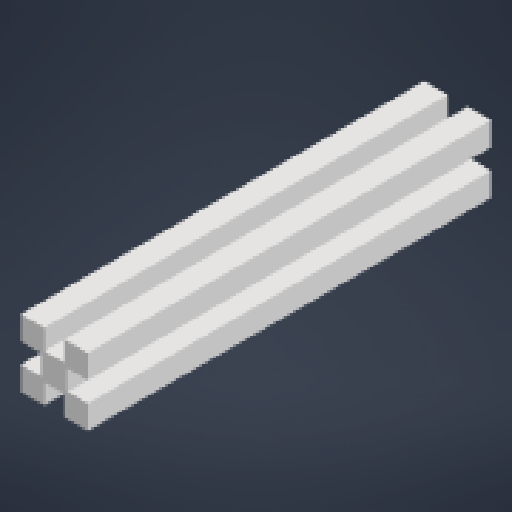
# Autodesk Inventor part: zbar
Saved by Autodesk Inventor 2025.1 (Build 291241020, 241B)
## iProperties
Created: 2024-09-23
Part Number: zbar
Material: Generic
Document SubType Name: Modeling
Designer: techn
Density: 1 g/cm^3
Appearance: Default
Author: techn
Autodesk Inventor part; units mm, degrees
ref_plane "YZ Plane" through (0, 0, 0) normal (1, 0, 0) x (0, 1, 0)
ref_plane "XZ Plane" through (0, 0, 0) normal (0, 1, 0) x (-1, 0, 0)
ref_plane "XY Plane" through (0, 0, 0) normal (0, 0, 1) x (1, 0, 0)
sketch "Sketch1" plane through (0, 0, 0) normal (0, 0, 1) x (1, 0, 0)
  line L0 (18, 7) -> (-162, 7) projected
  line L1 (-162, 0) -> (-162, 7) projected
  line L2 (18, 0) -> (-162, 0) projected
  line L3 (18, 7) -> (18, 0) projected
  line L4 (18, -6) -> (-162, -6) projected
  line L5 (-162, -13) -> (-162, -6) projected
  line L6 (-162, -13) -> (18, -13) projected
  line L7 (18, -6) -> (18, -13) projected
  line L8 (18, 0) -> (18, -6) projected
  line L9 (18, 7) -> (11, 7)
  line L10 (11, 7) -> (11, 0)
  line L11 (11, 0) -> (18, 0)
  line L12 (18, 0) -> (18, 7)
  line L13 (18, -6) -> (11, -6)
  line L14 (11, -6) -> (11, -13)
  line L15 (11, -13) -> (18, -13)
  line L16 (18, -13) -> (18, -6)
  line L17 (5, -13) -> (-2, -13)
  line L18 (-2, -13) -> (-2, -6)
  line L19 (-2, -6) -> (5, -6)
  line L20 (5, -6) -> (5, -13)
  line L21 (5, 0) -> (-2, 0)
  line L22 (-2, 0) -> (-2, 7)
  line L23 (-2, 7) -> (5, 7)
  line L24 (5, 7) -> (5, 0)
  line L25 (12, 1) -> (4, 1)
  line L26 (4, 1) -> (4, -7)
  line L27 (4, -7) -> (12, -7)
  line L28 (12, -7) -> (12, 1)
  point P0 (0, 0)
  point P1 (12, 0)
  point P2 (11, 1)
  point P3 (5, 1)
  point P4 (-2, 0)
  point P5 (4, 0)
  point P6 (4, -6)
  point P7 (-2, -13)
  point P8 (5, -7)
  point P9 (11, -7)
  point P10 (12, -6)
  dimension "d0" = 7
  dimension "d1" = 7
  dimension "d2" = 7
  dimension "d3" = 7
  dimension "d4" = 7
  dimension "d5" = 7
  dimension "d6" = 7
  dimension "d7" = 7
  dimension "d8" = 6
  dimension "d9" = 8
  dimension "d10" = 8
  dimension "d11" = 1
  dimension "d12" = 1
  constraints: 40 end point, 10 parallel, 5 horizontal, 5 perpendicular, 3 point on line
  measures "d0" distance of L11.end L10.end
  measures "d1" distance of L10.end L9.end
  measures "d2" distance of L15.end L14.end
  measures "d3" distance of L14.end L13.end
  measures "d4" distance of L18.end L19.end
  measures "d5" distance of L17.end L18.end
  measures "d6" distance of L22.end L23.end
  measures "d7" distance of L21.end L22.end
  measures "d8" distance between parallel lines of L24 L10
  measures "d9" distance of L27.end L26.end
  measures "d10" distance of L26.end L25.end
  measures "d11" distance between parallel lines of L27 L4
  measures "d12" distance between parallel lines of L14 L28
extrude "Extrusion1" add sketch "Sketch1" along normal blind 120 contours L3 L2 L28 L25 L10 L0 | L24 L25 L26 L2 L22 L0 | L25 L28 L2 L10 | L10 L2 L24 L25 | L28 L4 L26 L2 | L7 L6 L14 L27 L28 L4 | L24 L2 L26 L25 | L28 L27 L14 L4 | L14 L27 L20 L4 | L20 L27 L26 L4 | L6 L18 L4 L26 L27 L20
body "Solid1"
